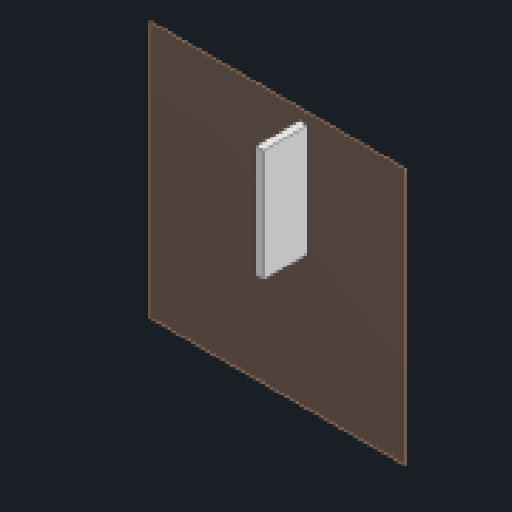
# Autodesk Inventor part: left_gear_holder
Saved by Autodesk Inventor 2023 (Build 270158000, 158)
## iProperties
Created: 2024-04-23
Part Number: left_gear_holder
Material: Generic
Document SubType Name: Modeling
Designer: szymo
Density: 1 g/cm^3
Appearance: Default
Author: szymo
Autodesk Inventor part; units mm, degrees
ref_plane "YZ Plane" through (0, 0, 0) normal (1, 0, 0) x (0, 1, 0)
ref_plane "XZ Plane" through (0, 0, 0) normal (0, 1, 0) x (-1, 0, 0)
ref_plane "Work Plane1" through (0, 0, 0) normal (0, 0, 1) x (1, 0, 0)
sketch "Sketch1" plane through (0, 0, 0) normal (0, 0, 1) x (1, 0, 0)
  line L0 (23.5, 89.5) -> (-23.5, 89.5) projected
  line L1 (-23.5, 89.5) -> (-23.5, 37.5) projected
  arc A0 (-26.5, 34.5) -> (-23.5, 37.5) centre (-26.5, 37.5) ccw projected
  line L2 (-26.5, 34.5) -> (-89, 34.5) projected
  line L3 (-89, 34.5) -> (-89, -69.5) projected
  line L4 (-89, -69.5) -> (-77, -69.5) projected
  arc A1 (-74, -72.5) -> (-77, -69.5) centre (-77, -72.5) ccw projected
  line L5 (-74, -72.5) -> (-74, -89.5) projected
  line L6 (-74, -89.5) -> (74, -89.5) projected
  line L7 (74, -89.5) -> (74, -72.5) projected
  arc A2 (77, -69.5) -> (74, -72.5) centre (77, -72.5) ccw projected
  line L8 (77, -69.5) -> (89, -69.5) projected
  line L9 (89, -69.5) -> (89, 34.5) projected
  line L10 (89, 34.5) -> (26.5, 34.5) projected
  arc A3 (23.5, 37.5) -> (26.5, 34.5) centre (26.5, 37.5) ccw projected
  line L11 (23.5, 37.5) -> (23.5, 89.5) projected
  line L12 (-4.5, 82.5) -> (-4.5, 37.5) projected
  arc A4 (-7.5, 34.5) -> (-4.5, 37.5) centre (-7.5, 37.5) ccw projected
  line L13 (-7.5, 34.5) -> (-13.5, 34.5) projected
  arc A5 (-16.5, 37.5) -> (-13.5, 34.5) centre (-13.5, 37.5) ccw projected
  line L14 (-16.5, 37.5) -> (-16.5, 82.5) projected
  arc A6 (-13.5, 85.5) -> (-16.5, 82.5) centre (-13.5, 82.5) ccw projected
  line L15 (-13.5, 85.5) -> (-7.5, 85.5) projected
  arc A7 (-4.5, 82.5) -> (-7.5, 85.5) centre (-7.5, 82.5) ccw projected
  line L16 (16.5, 82.5) -> (16.5, 37.5) projected
  arc A8 (13.5, 34.5) -> (16.5, 37.5) centre (13.5, 37.5) ccw projected
  line L17 (13.5, 34.5) -> (7.5, 34.5) projected
  arc A9 (4.5, 37.5) -> (7.5, 34.5) centre (7.5, 37.5) ccw projected
  line L18 (4.5, 37.5) -> (4.5, 82.5) projected
  arc A10 (7.5, 85.5) -> (4.5, 82.5) centre (7.5, 82.5) ccw projected
  line L19 (7.5, 85.5) -> (13.5, 85.5) projected
  arc A11 (16.5, 82.5) -> (13.5, 85.5) centre (13.5, 82.5) ccw projected
  line L20 (16.5, 89.5) -> (22.5, 89.5)
  line L21 (22.5, 89.5) -> (22.5, 3.75)
  line L22 (22.5, 3.75) -> (16.5, 3.75)
  line L23 (16.5, 3.75) -> (16.5, 89.5)
  line L24 (59.9, 4.75) -> (32.2, 4.75)
  point P0 (0, 0)
  dimension "d0" = 1
  dimension "d1" = 1
  constraints: 10 end point, 2 horizontal, 2 parallel, 1 collinear, 1 perpendicular, 1 point on line, 2 other
  measures "d0" distance between parallel lines of L21 L11
  measures "d1" distance between parallel lines of L24 L22
ref_plane "Work Plane2" through (-89, -40.3889, 33.5) normal (0, 0, 1) x (1, 0, 0)
extrude "Extrusion1" add sketch "Sketch1" along normal up to surface (33.5 mm away) contours L21 L22 L23 L16 L0
body "Solid1"
